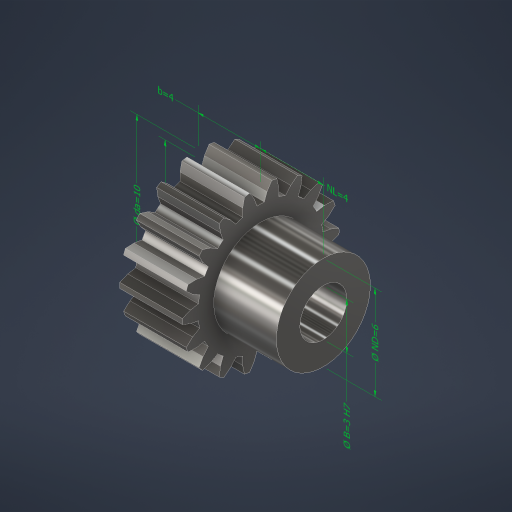
# Autodesk Inventor part: 18z
Saved by Autodesk Inventor 2024.1 (Build 281209000, 209)
## iProperties
Category: PARTsolutions
Company: MAEDLER
Created: 2023-10-16
Part Number: 18z
Material: Generic
Catalog Web Link: www.cadenas.de
Description: MAE-STZR-M0.5-MN-B4-ST-Spur Gears Made from Steel (11SMNPb30), with One-Sided Hub, Module 0.5, Tooth Width 4 mm
Vendor: MAEDLER
Document SubType Name: Modeling
Designer: psAdmin
Manufacturer: MAEDLER
Mass: 2 g
Surface Area: 4.73997 cm^2
Volume: 0.307298 cm^3
Density: 1 g/cm^3
Appearance: Stahl - poliert
PSOL_IDENT_0: {$CADENAS_DATA/23d-libs/maedler/antriebselemente/stirnzahnraeder/stirnzahnraeder_stahl/modul_0_5_und
PSOL_IDENT_1: _0_7/stzr_m_0_5_zb4_st_mn.prj},172 {VTYP=3D},{NB=21101800},{LINA=21101800},{NN=MAE-STZR-M0.5-MN-B4-S
PSOL_IDENT_2: T},{DATE=23.07.2023 13:56:16},{GEOMDATE=23.07.2023 13:56:16},{VERSION=},{LINEID=80},{WBVAR=},{WBNUME
PSOL_IDENT_3: RIC=}  {NB=21101800},{LINA=21101800},{KT=DUMMY},{ARTNR=21101800},{WEBSHOP=Produktdetails / Katalogse
PSOL_IDENT_4: ite / Montageanleitung},{MAT=Stahl 11SMnPb30+SH (1.0718)},{M=0.5},{Z=18},{B=4},{DA=10.0},{D=9.0},{NL=
PSOL_IDENT_5: 4},{ND=6},{BH7=3},{MD=1.7},{GEW=2.0},{ZTN=84839089},{DIST=0.600}
NB: 21101800
NN: MAE-STZR-M0.5-MN-B4-ST
NT: Spur Gears Made from Steel (11SMNPb30), with One-Sided Hub, Module 0.5, Tooth Width 4 mm
NBSYN: $ARTNR.
LINA: 21101800
CATALOG: Mädler
ARTNR: 21101800
WEBSHOP: Product details / Catalogue page / Assembly instructions
MAT: Steel 11SMnPb30+SH (1.0718)
M: 0.5
Z: 18
B: 4
DA: 10
D: 9
NL: 4
ND: 6
BH7: 3
MD: 1.7
GEW: 2
ZTN: 84839089
SUPPLIER: MAEDLER
ARTICLENO: 21101800
BOMINFO: 21101800
CREATOR: CADENAS GmbH
Title: 21101800
Author: Cadenas PARTsolutions
Comments: Spur Gears Made from Steel (11SMNPb30), with One-Sided Hub, Module 0.5, Tooth Width 4 mm
Autodesk Inventor part; units mm, degrees
ref_plane "YZ Plane" through (0, 0, 0) normal (1, 0, 0) x (0, 1, 0)
ref_plane "XZ Plane" through (0, 0, 0) normal (0, 1, 0) x (-1, 0, 0)
ref_plane "XY Plane" through (0, 0, 0) normal (0, 0, 1) x (1, 0, 0)
sketch "Skizze_1" plane through (0, 0, 0) normal (1, 0, 0) x (0, 1, 0)
  arc A0 (0.1667, 4.9972) -> (-0.1667, 4.9972) centre (0, 0) ccw
  line L0 (-0.1667, 4.9972) -> (-0.3742, 4.4844)
  line L1 (-0.3742, 4.4844) -> (-0.4644, 3.973)
  arc A1 (-0.4644, 3.973) -> (-0.9225, 3.8922) centre (0, 0) ccw
  line L2 (-0.9225, 3.8922) -> (-1.1821, 4.342)
  line L3 (-1.1821, 4.342) -> (-1.5525, 4.7529)
  arc A2 (-1.5525, 4.7529) -> (-1.8658, 4.6388) centre (0, 0) ccw
  line L4 (-1.8658, 4.6388) -> (-1.8854, 4.086)
  line L5 (-1.8854, 4.086) -> (-1.7952, 3.5745)
  arc A3 (-1.7952, 3.5745) -> (-2.198, 3.342) centre (0, 0) ccw
  line L6 (-2.198, 3.342) -> (-2.5959, 3.6758)
  line L7 (-2.5959, 3.6758) -> (-3.0845, 3.9352)
  arc A4 (-3.0845, 3.9352) -> (-3.3398, 3.721) centre (0, 0) ccw
  line L8 (-3.3398, 3.721) -> (-3.1692, 3.1947)
  line L9 (-3.1692, 3.1947) -> (-2.9095, 2.745)
  arc A5 (-2.9095, 2.745) -> (-3.2085, 2.3886) centre (0, 0) ccw
  line L10 (-3.2085, 2.3886) -> (-3.6965, 2.5663)
  line L11 (-3.6965, 2.5663) -> (-4.2444, 2.6429)
  arc A6 (-4.2444, 2.6429) -> (-4.4111, 2.3543) centre (0, 0) ccw
  line L12 (-4.4111, 2.3543) -> (-4.0707, 1.9182)
  line L13 (-4.0707, 1.9182) -> (-3.6729, 1.5843)
  arc A7 (-3.6729, 1.5843) -> (-3.832, 1.1472) centre (0, 0) ccw
  line L14 (-3.832, 1.1472) -> (-4.3513, 1.1472)
  line L15 (-4.3513, 1.1472) -> (-4.8924, 1.0319)
  arc A8 (-4.8924, 1.0319) -> (-4.9502, 0.7036) centre (0, 0) ccw
  line L16 (-4.9502, 0.7036) -> (-4.4813, 0.4102)
  line L17 (-4.4813, 0.4102) -> (-3.9932, 0.2326)
  arc A9 (-3.9932, 0.2326) -> (-3.9932, -0.2326) centre (0, 0) ccw
  line L18 (-3.9932, -0.2326) -> (-4.4813, -0.4102)
  line L19 (-4.4813, -0.4102) -> (-4.9502, -0.7036)
  arc A10 (-4.9502, -0.7036) -> (-4.8924, -1.0319) centre (0, 0) ccw
  line L20 (-4.8924, -1.0319) -> (-4.3513, -1.1472)
  line L21 (-4.3513, -1.1472) -> (-3.832, -1.1472)
  arc A11 (-3.832, -1.1472) -> (-3.6729, -1.5843) centre (0, 0) ccw
  line L22 (-3.6729, -1.5843) -> (-4.0707, -1.9182)
  line L23 (-4.0707, -1.9182) -> (-4.4111, -2.3543)
  arc A12 (-4.4111, -2.3543) -> (-4.2444, -2.6429) centre (0, 0) ccw
  line L24 (-4.2444, -2.6429) -> (-3.6965, -2.5663)
  line L25 (-3.6965, -2.5663) -> (-3.2085, -2.3886)
  arc A13 (-3.2085, -2.3886) -> (-2.9095, -2.745) centre (0, 0) ccw
  line L26 (-2.9095, -2.745) -> (-3.1692, -3.1947)
  line L27 (-3.1692, -3.1947) -> (-3.3398, -3.721)
  arc A14 (-3.3398, -3.721) -> (-3.0845, -3.9352) centre (0, 0) ccw
  line L28 (-3.0845, -3.9352) -> (-2.5959, -3.6758)
  line L29 (-2.5959, -3.6758) -> (-2.198, -3.342)
  arc A15 (-2.198, -3.342) -> (-1.7952, -3.5745) centre (0, 0) ccw
  line L30 (-1.7952, -3.5745) -> (-1.8854, -4.086)
  line L31 (-1.8854, -4.086) -> (-1.8658, -4.6388)
  arc A16 (-1.8658, -4.6388) -> (-1.5525, -4.7529) centre (0, 0) ccw
  line L32 (-1.5525, -4.7529) -> (-1.1821, -4.342)
  line L33 (-1.1821, -4.342) -> (-0.9225, -3.8922)
  arc A17 (-0.9225, -3.8922) -> (-0.4644, -3.973) centre (0, 0) ccw
  line L34 (-0.4644, -3.973) -> (-0.3742, -4.4844)
  line L35 (-0.3742, -4.4844) -> (-0.1667, -4.9972)
  arc A18 (-0.1667, -4.9972) -> (0.1667, -4.9972) centre (0, 0) ccw
  line L36 (0.1667, -4.9972) -> (0.3742, -4.4844)
  line L37 (0.3742, -4.4844) -> (0.4644, -3.973)
  arc A19 (0.4644, -3.973) -> (0.9225, -3.8922) centre (0, 0) ccw
  line L38 (0.9225, -3.8922) -> (1.1821, -4.342)
  line L39 (1.1821, -4.342) -> (1.5525, -4.7529)
  arc A20 (1.5525, -4.7529) -> (1.8658, -4.6388) centre (0, 0) ccw
  line L40 (1.8658, -4.6388) -> (1.8854, -4.086)
  line L41 (1.8854, -4.086) -> (1.7952, -3.5745)
  arc A21 (1.7952, -3.5745) -> (2.198, -3.342) centre (0, 0) ccw
  line L42 (2.198, -3.342) -> (2.5959, -3.6758)
  line L43 (2.5959, -3.6758) -> (3.0845, -3.9352)
  arc A22 (3.0845, -3.9352) -> (3.3398, -3.721) centre (0, 0) ccw
  line L44 (3.3398, -3.721) -> (3.1692, -3.1947)
  line L45 (3.1692, -3.1947) -> (2.9095, -2.745)
  arc A23 (2.9095, -2.745) -> (3.2085, -2.3886) centre (0, 0) ccw
  line L46 (3.2085, -2.3886) -> (3.6965, -2.5663)
  line L47 (3.6965, -2.5663) -> (4.2444, -2.6429)
  arc A24 (4.2444, -2.6429) -> (4.4111, -2.3543) centre (0, 0) ccw
  line L48 (4.4111, -2.3543) -> (4.0707, -1.9182)
  line L49 (4.0707, -1.9182) -> (3.6729, -1.5843)
  arc A25 (3.6729, -1.5843) -> (3.832, -1.1472) centre (0, 0) ccw
  line L50 (3.832, -1.1472) -> (4.3513, -1.1472)
  line L51 (4.3513, -1.1472) -> (4.8924, -1.0319)
  arc A26 (4.8924, -1.0319) -> (4.9502, -0.7036) centre (0, 0) ccw
  line L52 (4.9502, -0.7036) -> (4.4813, -0.4102)
  line L53 (4.4813, -0.4102) -> (3.9932, -0.2326)
  arc A27 (3.9932, -0.2326) -> (3.9932, 0.2326) centre (0, 0) ccw
  line L54 (3.9932, 0.2326) -> (4.4813, 0.4102)
  line L55 (4.4813, 0.4102) -> (4.9502, 0.7036)
  arc A28 (4.9502, 0.7036) -> (4.8924, 1.0319) centre (0, 0) ccw
  line L56 (4.8924, 1.0319) -> (4.3513, 1.1472)
  line L57 (4.3513, 1.1472) -> (3.832, 1.1472)
  arc A29 (3.832, 1.1472) -> (3.6729, 1.5843) centre (0, 0) ccw
  line L58 (3.6729, 1.5843) -> (4.0707, 1.9182)
  line L59 (4.0707, 1.9182) -> (4.4111, 2.3543)
  arc A30 (4.4111, 2.3543) -> (4.2444, 2.6429) centre (0, 0) ccw
  line L60 (4.2444, 2.6429) -> (3.6965, 2.5663)
  line L61 (3.6965, 2.5663) -> (3.2085, 2.3886)
  arc A31 (3.2085, 2.3886) -> (2.9095, 2.745) centre (0, 0) ccw
  line L62 (2.9095, 2.745) -> (3.1692, 3.1947)
  line L63 (3.1692, 3.1947) -> (3.3398, 3.721)
  arc A32 (3.3398, 3.721) -> (3.0845, 3.9352) centre (0, 0) ccw
  line L64 (3.0845, 3.9352) -> (2.5959, 3.6758)
  line L65 (2.5959, 3.6758) -> (2.198, 3.342)
  arc A33 (2.198, 3.342) -> (1.7952, 3.5745) centre (0, 0) ccw
  line L66 (1.7952, 3.5745) -> (1.8854, 4.086)
  line L67 (1.8854, 4.086) -> (1.8658, 4.6388)
  arc A34 (1.8658, 4.6388) -> (1.5525, 4.7529) centre (0, 0) ccw
  line L68 (1.5525, 4.7529) -> (1.1821, 4.342)
  line L69 (1.1821, 4.342) -> (0.9225, 3.8922)
  arc A35 (0.9225, 3.8922) -> (0.4644, 3.973) centre (0, 0) ccw
  line L70 (0.4644, 3.973) -> (0.3742, 4.4844)
  line L71 (0.3742, 4.4844) -> (0.1667, 4.9972)
  constraints: 144 end point, 72 point on circle, 36 centre point
extrude "Extrusion1" add sketch "Skizze_1" along normal mid plane 4
sketch "Skizze_2" plane through (0, 0, 0) normal (0, 0, 1) x (1, 0, 0)
  line L0 (6, 0) -> (2, 0)
  line L1 (2, 0) -> (2, 3)
  line L2 (2, 3) -> (6, 3)
  line L3 (6, 3) -> (6, 0)
  line L4 (6, 0) -> (2, 0)
  constraints: 10 end point
revolve "Revolution1" add sketch "Skizze_2" angle 360 about axis through (6, 0, 0) along (1, 0, 0)
sketch "Skizze_3" plane through (6, 0, 0) normal (1, 0, 0) x (0, 1, 0)
  circle A0 centre (0, 0) radius 1.5
  constraints: 1 centre point
extrude "Extrusion2" cut sketch "Skizze_3" along normal mid plane 16
body "Solid1"
